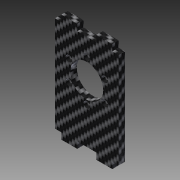
# Autodesk Inventor part: Motor Mount
Saved by Autodesk Inventor 2015 (Build 190159000, 159)
## iProperties
Created: 2016-09-19
Part Number: Motor Mount
Material: Generic
Document SubType Name: Modeling
Designer: James Yelland
Density: 1 g/cm^3
Appearance: Default
Author: James Yelland
Autodesk Inventor part; units mm, degrees
ref_plane "YZ Plane" through (0, 0, 0) normal (1, 0, 0) x (0, 1, 0)
ref_plane "XZ Plane" through (0, 0, 0) normal (0, 1, 0) x (-1, 0, 0)
ref_plane "XY Plane" through (0, 0, 0) normal (0, 0, 1) x (1, 0, 0)
sketch "Sketch1" plane through (0, 0, 0) normal (0, 1, 0) x (-1, 0, 0)
  circle A0 centre (0, 0) radius 5.15
  line L0 (10, -18) -> (8, -18)
  line L1 (8, -18) -> (8, -20)
  line L2 (8, -20) -> (3, -20)
  line L3 (3, -20) -> (3, -18)
  line L4 (3, -18) -> (-3, -18)
  line L5 (-3, -18) -> (-3, -20)
  line L6 (-3, -20) -> (-8, -20)
  line L7 (-8, -20) -> (-8, -18)
  line L8 (-8, -18) -> (-10, -18)
  line L9 (10, -18) -> (10, 12)
  line L10 (-10, -18) -> (-10, 12)
  line L11 (10, 12) -> (8, 12)
  line L12 (8, 12) -> (8, 14)
  line L13 (8, 14) -> (3, 14)
  line L14 (3, 14) -> (3, 12)
  line L15 (3, 12) -> (-3, 12)
  line L16 (-3, 12) -> (-3, 14)
  line L17 (-3, 14) -> (-8, 14)
  line L18 (-8, 14) -> (-8, 12)
  line L19 (-8, 12) -> (-10, 12)
  line L20 (0, 0) -> (0, 6.5)
  circle A1 centre (0, 6.5) radius 1
  circle A2 centre (-5.6292, 3.25) radius 1
  circle A3 centre (-5.6292, -3.25) radius 1
  circle A4 centre (0, -6.5) radius 1
  circle A5 centre (5.6292, -3.25) radius 1
  circle A6 centre (5.6292, 3.25) radius 1
  dimension "d7" = 360
  dimension "d33" = 2
  dimension "d34" = 2
  dimension "d35" = 5
  dimension "d36" = 6
  dimension "d37" = 5
  dimension "d42" = 30
  dimension "d43" = 2
  dimension "d44" = 2
  dimension "d45" = 5
  dimension "d46" = 6
  dimension "d47" = 5
  dimension "d48" = 6.5
  dimension "d49" = 2
  dimension "d52" = 360
  constraints: 42 end point, 12 perpendicular, 10 point on line, 7 centre point, 3 vertical, 2 coincident, 2 horizontal, 14 other
  measures "d33" distance of L0.start L0.end
  measures "d34" distance of L0.end L1.end
  measures "d35" distance of L1.end L2.end
  measures "d36" distance of L3.end L4.end
  measures "d37" distance of L5.end L6.end
  measures "d42" distance of L8.end L10.end
  measures "d43" distance of L9.end L11.end
  measures "d44" distance of L11.end L12.end
  measures "d45" distance of L12.end L13.end
  measures "d46" distance of L14.end L15.end
  measures "d47" distance of L16.end L17.end
  measures "d48" distance of L20.start L20.end
  measures "d49" diameter of A1
extrude "Extrusion1" add sketch "Sketch1" along normal blind 2
body "Solid1"
